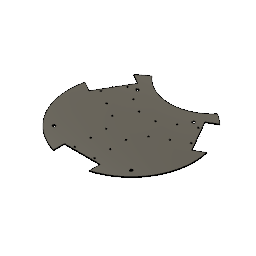
Plate_Bot (Autodesk Fusion 360 design; units mm, degrees)
Autodesk Fusion 360 part; units mm, degrees
note: some values were not read from the file. Set by a fixed rule: which sketch regions a step uses.
sketch "Esboço1" plane through (0, 0, 0) normal (0, 0, 1) x (1, 0, 0)
  circle A0 centre (0, 0) radius 240
  circle A1 centre (148, -148) radius 5
  line L0 (-125, 204.878) -> (125, 204.878)
  circle A2 centre (0, 311.043) radius 164
  circle A3 centre (107.5, 130.5) radius 5
  line L1 (-40, 115) -> (40, 115)
  line L2 (-40, 115) -> (-40, 151.9958)
  line L3 (40, 115) -> (40, 151.9958)
  line L4 (0, 1.75) -> (0, 22.5)
  circle A4 centre (-148, -148) radius 5
  circle A5 centre (-107.5, 130.5) radius 5
  line L5 (-68, -188) -> (68, -188)
  line L6 (68, -188) -> (68, -240)
  line L7 (68, -240) -> (-68, -240)
  line L8 (-68, -240) -> (-68, -188)
  line L9 (0, -188) -> (0, -178)
  line L10 (-37.5, -178) -> (37.5, -178)
  circle A6 centre (-37.5, -178) radius 2.5
  circle A7 centre (37.5, -178) radius 2.5
  circle A8 centre (37.5, -118) radius 2.5
  circle A9 centre (37.5, -58) radius 2.5
  circle A10 centre (-37.5, -118) radius 2.5
  circle A11 centre (-37.5, -58) radius 2.5
  circle A12 centre (135.4025, 121.476) radius 2.5
  line L11 (241.8461, 61.1103) -> (196.8128, 35.1103)
  line L12 (196.8128, 35.1103) -> (128.8128, 152.8897)
  line L13 (128.8128, 152.8897) -> (173.8461, 178.8897)
  circle A13 centre (83.441, 91.476) radius 2.5
  circle A14 centre (172.9025, 56.524) radius 2.5
  circle A15 centre (120.941, 26.524) radius 2.5
  circle A16 centre (68.9795, -3.476) radius 2.5
  circle A17 centre (31.4795, 61.476) radius 2.5
  circle A18 centre (-172.9025, 56.524) radius 2.5
  line L14 (-173.8461, 178.8897) -> (-128.8128, 152.8897)
  line L15 (-128.8128, 152.8897) -> (-196.8128, 35.1103)
  line L16 (-196.8128, 35.1103) -> (-241.8461, 61.1103)
  circle A19 centre (-120.941, 26.524) radius 2.5
  circle A20 centre (-135.4025, 121.476) radius 2.5
  circle A21 centre (-83.441, 91.476) radius 2.5
  circle A22 centre (-31.4795, 61.476) radius 2.5
  circle A23 centre (-68.9795, -3.476) radius 2.5
  point P0 (0, 115)
  point P1 (0, -240)
  point P2 (-68, -230.1652)
  dimension "d1" = 480
  dimension "d13" = 10
  dimension "d14" = 148
  dimension "d15" = 148
  dimension "d16" = 250
  dimension "d17" = 328
  dimension "d18" = 10
  dimension "d19" = 130.5
  dimension "d20" = 107.5
  dimension "d21" = 115
  dimension "d22" = 80
  dimension "d25" = 136
  dimension "d26" = 52
  dimension "d27" = 10
  dimension "d28" = 75
  dimension "d29" = 5
  dimension "d30" = 5
  dimension "d33" = 1
  dimension "d34" = 60
  dimension "d36" = 360
  constraint coincident A0.centre origin
  constraint horizontal L0
  constraint coincident A0 L0.start
  constraint coincident A0 L0.end
  constraint coincident L0.start A2
  constraint coincident L0.end A2
  constraint horizontal L1
  constraint midpoint P0 L1
  constraint coincident A2 L2.end
  constraint perpendicular L1 L2
  constraint coincident A2 L3.end
  constraint perpendicular L1 L3
  constraint symmetric A1 L4 A4
  constraint symmetric A3 L4 A5
  constraint horizontal L5
  constraint vertical L6
  constraint horizontal L7
  constraint vertical L8
  constraint midpoint L7 P1
  constraint tangent A0 L7
  constraint coincident A0 P1
  constraint midpoint L5 L9.start
  constraint perpendicular L5 L9
  constraint horizontal L10
  constraint midpoint L9.end L10
  constraint coincident L10.start A6.centre
  constraint coincident L10.end A7.centre
  constraint coincident A0 P2
  constraint coincident L8 P2
  measures "d1" diameter of A0
  measures "d13" diameter of A1
  measures "d14" vertical distance of A0.centre A1.centre
  measures "d15" horizontal distance of A0.centre A1.centre
  measures "d16" distance of L0.start L0.end
  measures "d17" diameter of A2
  measures "d18" diameter of A3
  measures "d19" vertical distance of A0.centre A3.centre
  measures "d20" horizontal distance of A0.centre A3.centre
  measures "d21" distance of A0.centre P0
  measures "d22" distance of L1.start L1.end
  measures "d25" distance of L5.start L5.end
  measures "d26" distance of L5.start L7.end
  measures "d27" distance of L9.start L9.end
  measures "d28" distance of L10.start L10.end
  measures "d29" diameter of A6
  measures "d30" diameter of A7
extrude "Extrusão1" add sketch "Esboço1" along normal blind 3 contours A0 A2 L1 L2 L3 L5 L6 L8 L11 L12 L13 L14 L15 L16 | A2 L1 L2 L3
sketch "Esboço2" plane through (162.8128, 94, 0) normal (0.866025, 0.5, 0) x (-0.5, 0.866025, 0)
  line L0 (-68, 0) -> (68, 0)
  line L1 (68, 0) -> (68, 3)
  line L2 (68, 3) -> (-68, 3)
  line L3 (-68, 3) -> (-68, 0)
  line L4 (68, 0) -> (-68, 0)
  line L5 (-68, 0) -> (-68, 3)
  line L6 (-68, 3) -> (68, 3)
  line L7 (68, 3) -> (68, 0)
  line L8 (0, 0) -> (0, 3) construction
  line L9 (-68, 1.5) -> (68, 1.5) construction
  circle A0 centre (0, 1.5) radius 0.75
  dimension "d38" = 1.5
  constraint horizontal L4
  constraint vertical L5
  constraint horizontal L6
  constraint vertical L7
  constraint coincident L2.end L3.start
  constraint coincident L0.end L1.start
  constraint coincident L8.start origin
  constraint midpoint L2 L8.end
  constraint midpoint L3 L9.start
  constraint midpoint L1 L9.end
  constraint midpoint L9 A0.centre
  measures "d38" diameter of A0
sketch "Esboço3" plane through (0, -188, 0) normal (0, -1, 0) x (1, 0, 0)
  line L0 (-68, 0) -> (68, 0)
  line L1 (68, 0) -> (68, 3)
  line L2 (68, 3) -> (-68, 3)
  line L3 (-68, 3) -> (-68, 0)
  line L4 (68, 0) -> (-68, 0)
  line L5 (-68, 0) -> (-68, 3)
  line L6 (-68, 3) -> (68, 3)
  line L7 (68, 3) -> (68, 0)
  line L8 (0, 0) -> (0, 3) construction
  line L9 (-68, 1.5) -> (68, 1.5) construction
  circle A0 centre (0, 1.5) radius 0.75
  dimension "d39" = 1.5
  constraint horizontal L4
  constraint vertical L5
  constraint horizontal L6
  constraint vertical L7
  constraint coincident L2.end L3.start
  constraint coincident L0.end L1.start
  constraint coincident L8.start origin
  constraint midpoint L2 L8.end
  constraint midpoint L3 L9.start
  constraint midpoint L1 L9.end
  constraint midpoint L8 A0.centre
  measures "d39" diameter of A0
sketch "Esboço4" plane through (-162.8128, 94, 0) normal (-0.866025, 0.5, 0) x (-0.5, -0.866025, 0)
  line L0 (-68, 0) -> (68, 0)
  line L1 (68, 0) -> (68, 3)
  line L2 (68, 3) -> (-68, 3)
  line L3 (-68, 3) -> (-68, 0)
  line L4 (68, 0) -> (-68, 0)
  line L5 (-68, 0) -> (-68, 3)
  line L6 (-68, 3) -> (68, 3)
  line L7 (68, 3) -> (68, 0)
  line L8 (0, 0) -> (0, 3) construction
  line L9 (68, 1.5) -> (-68, 1.5) construction
  circle A0 centre (0, 1.5) radius 0.75
  dimension "d40" = 1.5
  constraint horizontal L4
  constraint vertical L5
  constraint horizontal L6
  constraint vertical L7
  constraint coincident L2.end L3.start
  constraint coincident L0.end L1.start
  constraint coincident L8.start origin
  constraint midpoint L2 L8.end
  constraint midpoint L1 L9.start
  constraint midpoint L3 L9.end
  constraint midpoint L9 A0.centre
  measures "d40" diameter of A0
extrude "Extrusão2" add sketch "Esboço4" along normal blind 5 contours A0
extrude "Extrusão3" add sketch "Esboço2" along normal blind 5 contours A0
extrude "Extrusão4" add sketch "Esboço3" along normal blind 5 contours A0
equation "d17 = ( 164 * 2 ) * 1 mm"
